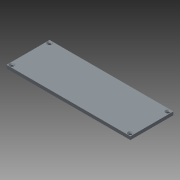
# Autodesk Inventor part: 13_1087_024
Saved by Autodesk Inventor 2014 (Build 180170000, 170)
## iProperties
Created: 2013-09-11
Part Number: 13_1087_024
Material: Allgemein
Document SubType Name: Modeling
Designer: vogel
Density: 1 g/cm^3
Appearance: Zink
Author: vogel
Autodesk Inventor part; units mm, degrees
ref_plane "YZ Plane" through (0, 0, 0) normal (1, 0, 0) x (0, 1, 0)
ref_plane "XZ Plane" through (0, 0, 0) normal (0, 1, 0) x (-1, 0, 0)
ref_plane "XY Plane" through (0, 0, 0) normal (0, 0, 1) x (1, 0, 0)
sketch "Skizze1" plane through (0, 0, 0) normal (0, 0, 1) x (1, 0, 0)
  line L0 (-23, 0) -> (138, 0) projected
  line L1 (0, -8) -> (0, 48) projected
  line L2 (0, 0) -> (115, 0)
  line L3 (115, 0) -> (115, 40)
  line L4 (115, 40) -> (0, 40)
  line L5 (0, 40) -> (0, 0)
  dimension "d0" = 40
  dimension "d1" = 115
  constraints: 8 end point, 2 parallel, 1 horizontal, 1 perpendicular
  measures "d0" distance of L4.end L2.start
  measures "d1" distance of L2.start L2.end
extrude "Extrusion1" add sketch "Skizze1" along normal blind 3
sketch "Skizze2" plane through (0, 0, 3) normal (0, 0, 1) x (1, 0, 0)
  line L0 (0, 0) -> (115, 0) projected
  line L1 (115, 0) -> (115, 40) projected
  line L2 (115, 40) -> (0, 40) projected
  line L3 (0, 40) -> (0, 0) projected
  line L4 (2.5, 37.5) -> (112.5, 37.5)
  line L5 (112.5, 37.5) -> (112.5, 2.5)
  line L6 (112.5, 2.5) -> (2.5, 2.5)
  line L7 (2.5, 2.5) -> (2.5, 37.5)
  dimension "d5" = 2.5
  constraints: 8 end point, 4 coincident, 3 other
  measures "d5" distance between parallel lines of L2 L4
hole "Bohrung1" at (2.5, 37.5, 3) at (2.5, 2.5, 3) at (112.5, 2.5, 3) at (112.5, 37.5, 3) direction (0, 0, -1) diameter 2.4 end through all countersink diameter 4.5 countersink angle 90
